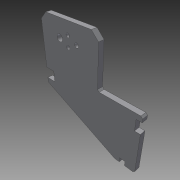
# Autodesk Inventor part: z_axis_top
Saved by Autodesk Inventor 2014 (Build 180170000, 170)
## iProperties
Created: 2014-03-30
Part Number: z_axis_top
Material: Generic
Document SubType Name: Modeling
Designer: buben
Density: 1 g/cm^3
Appearance: Default
Author: buben
Autodesk Inventor part; units mm, degrees
ref_plane "YZ Plane" through (0, 0, 0) normal (1, 0, 0) x (0, 1, 0)
ref_plane "XZ Plane" through (0, 0, 0) normal (0, 1, 0) x (-1, 0, 0)
ref_plane "XY Plane" through (0, 0, 0) normal (0, 0, 1) x (1, 0, 0)
sketch "Sketch1" plane through (0, 0, 0) normal (0, 1, 0) x (-1, 0, 0)
  line L0 (0, -6) -> (0, 0)
  line L1 (0, 0) -> (-12, 0)
  line L2 (-12, 0) -> (-12, 13)
  line L3 (-12, 13) -> (0, 13)
  line L4 (0, 13) -> (0, 67)
  line L5 (0, 67) -> (-8, 75)
  line L6 (-8, 75) -> (-67, 75)
  line L7 (-67, 75) -> (-75, 67)
  line L8 (0, -6) -> (-100, -50)
  line L9 (-100, -50) -> (-124.5, -50)
  line L10 (-124.5, -50) -> (-124.5, 0)
  line L11 (-124.5, 0) -> (-118.5, 0)
  line L12 (-118.5, 0) -> (-118.5, 13)
  line L13 (-118.5, 13) -> (-124.5, 13)
  line L14 (-124.5, 13) -> (-124.5, 19)
  line L15 (-124.5, 19) -> (-75, 19)
  line L16 (-75, 19) -> (-75, 67)
  circle A0 centre (-26, 55) radius 4
  circle A1 centre (-49, 55) radius 2.5
  line L17 (-106, -50) -> (-112.5, -50) construction
  line L18 (-112.5, -50) -> (-112.5, 13) construction
  line L19 (-112.5, 13) -> (-106, 13) construction
  line L20 (-106, 13) -> (-106, -50) construction
  dimension "d0" = 13
  dimension "d1" = 12
  dimension "d2" = 6
  dimension "d3" = 6
  dimension "d4" = 6
  dimension "d6" = 75
  dimension "d7" = 8
  dimension "d8" = 5
  dimension "d9" = 23
  dimension "d10" = 106.5
  dimension "d11" = 45
  dimension "d12" = 8
  dimension "d13" = 6.5
  dimension "d14" = 6
  dimension "d15" = 6
  dimension "d16" = 42
  dimension "d17" = 20
  dimension "d18" = 50
  dimension "d19" = 26
  constraints: 42 end point, 10 perpendicular, 7 collinear, 7 parallel, 2 centre point, 1 horizontal, 1 horizontal alignment, 1 vertical
  measures "d0" distance of L1.end L2.end
  measures "d1" distance of L0.end L1.end
  measures "d2" distance of L10.end L11.end
  measures "d3" distance of L0.start L0.end
  measures "d4" distance of L13.end L14.end
  measures "d6" distance between parallel lines of L16 L4
  measures "d7" diameter of A0
  measures "d8" diameter of A1
  measures "d9" distance of A1.centre A0.centre
  measures "d10" distance between parallel lines of L2 L12
  measures "d11" angle of L4 L5
  measures "d12" horizontal distance of L4.end L5.end
  measures "d13" distance of L18.end L19.end
  measures "d14" distance between parallel lines of L12 L18
  measures "d15" distance from line of L8.end L20
  measures "d16" distance from line of L3 A0.centre
  measures "d17" distance from line of L6 A0.centre
  measures "d18" distance between parallel lines of L9 L11
  measures "d19" distance from line of L4 A0.centre
extrude "Extrusion1" add sketch "Sketch1" along normal blind 6.5
sketch "Sketch3" plane through (0, 6.5, 0) normal (0, 1, 0) x (1, 0, 0)
  line L0 (124.5, 0) -> (124.5, 50) projected
  line L1 (124.5, 50) -> (100, 50) projected
  line L2 (106, 50) -> (112.5, 50)
  line L3 (112.5, 50) -> (112.5, 44)
  line L4 (112.5, 44) -> (106, 44)
  line L5 (106, 44) -> (106, 50)
  dimension "d27" = 6
  dimension "d28" = 6.5
  dimension "d29" = 12
  constraints: 8 end point, 2 parallel, 1 horizontal, 1 perpendicular, 1 point on line
  measures "d27" distance of L4.end L2.start
  measures "d28" distance of L3.end L4.end
  measures "d29" distance between parallel lines of L0 L3
extrude "Extrusion3" cut sketch "Sketch3" against normal through all
chamfer "Chamfer1" distance 2 angle 45 3 edges at (75, 3.25, 19) (124.5, 3.25, 19) (124.5, 3.25, -50)
sketch "Sketch4" plane through (0, 6.5, 0) normal (0, 1, 0) x (1, 0, 0)
  line L0 (124.5, 0) -> (124.5, 48) projected
  circle A0 centre (26, -55) radius 4 projected
  circle A1 centre (49, -55) radius 2.5 projected
  circle A2 centre (37.5, -49) radius 2.25
  circle A3 centre (37.5, -61) radius 2.25
  line L1 (37.5, -49) -> (37.5, -61) construction
  line L2 (26, -55) -> (49, -55) construction
  point P0 (37.5, -55)
  dimension "d35" = 12
  dimension "d36" = 4.5
  constraints: 4 end point, 2 centre point, 2 midpoint, 1 equal radius, 1 parallel, 1 perpendicular, 1 vertical alignment
  measures "d35" distance of L1.end L1.start
  measures "d36" diameter of A2
extrude "Extrusion4" cut sketch "Sketch4" against normal through all contours A2 | A3
equation "\"d2\" = d3"
equation "\"d4\" = d3"
body "Solid1"
